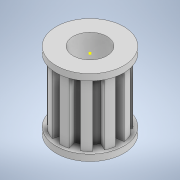
# Autodesk Inventor part: Pièce_moteur_courroie_test_1
Saved by Autodesk Inventor 2020.1 (Build 241239000, 239)
## iProperties
Created: 2019-07-26
Part Number: Pièce_moteur_courroie_test_1
Material: Générique
Document SubType Name: Modeling
Designer: marlo
Density: 1 g/cm^3
Appearance: Par défaut
Author: marlo
Autodesk Inventor part; units mm, degrees
ref_plane "YZ Plane" through (0, 0, 0) normal (1, 0, 0) x (0, 1, 0)
ref_plane "XZ Plane" through (0, 0, 0) normal (0, 1, 0) x (-1, 0, 0)
ref_plane "XY Plane" through (0, 0, 0) normal (0, 0, 1) x (1, 0, 0)
sketch "Esquisse2" plane through (0, 0, 0) normal (0, 1, 0) x (-1, 0, 0)
  circle A0 centre (0, 0) radius 7.2
  dimension "d0" = 14.4
  constraints: 1 centre point, 1 coincident
  measures "d0" diameter of A0
extrude "Extrusion1" add sketch "Esquisse2" along normal blind 15
sketch "Esquisse4" plane through (0, 15, 0) normal (0, 1, 0) x (1, 0, 0)
  circle A0 centre (0, 0) radius 7.2 projected
  circle A1 centre (0, 0) radius 7.2 projected
  arc A2 (-2, -6.9166) -> (0, -7.2) centre (0, 0) ccw
  arc A3 (-1.4444, -4.9954) -> (0, -5.2) centre (0, 0) ccw
  line L0 (-2, -6.9166) -> (-1.4444, -4.9954)
  line L1 (0, -7.2) -> (0, -5.2)
  line L2 (0, 0) -> (-4.1531, -9.129)
  arc A4 (-5.4277, -4.7308) -> (-3.9, -6.0523) centre (0, 0) ccw
  arc A5 (-3.92, -3.4167) -> (-2.8167, -4.3711) centre (0, 0) ccw
  line L3 (-3.9, -6.0523) -> (-2.8167, -4.3711)
  line L4 (-5.4277, -4.7308) -> (-3.92, -3.4167)
  line L5 (0, -6) -> (0, 5.5969) construction
  line L6 (0, 0) -> (-5.5895, -3.594)
  arc A6 (-6.5507, 2.988) -> (-7.1229, 1.0507) centre (0, 0) ccw
  arc A7 (-4.7311, 2.158) -> (-5.1443, 0.7589) centre (0, 0) ccw
  line L7 (-7.1229, 1.0507) -> (-5.1443, 0.7589)
  line L8 (-6.5507, 2.988) -> (-4.7311, 2.158)
  arc A8 (-7.125, -1.0366) -> (-6.5566, -2.975) centre (0, 0) ccw
  arc A9 (-5.1458, -0.7487) -> (-4.7353, -2.1486) centre (0, 0) ccw
  line L9 (-7.125, -1.0366) -> (-5.1458, -0.7487)
  line L10 (-6.5566, -2.975) -> (-4.7353, -2.1486)
  line L11 (-2, -6.9166) -> (-3.9, -6.0523) construction
  line L12 (-5.4277, -4.7308) -> (-6.5566, -2.975) construction
  line L13 (-2, -6.9166) -> (0, -7.2) construction
  line L14 (0, 0) -> (-5.7368, 3.7048)
  arc A10 (-3.888, 6.06) -> (-5.4183, 4.7415) centre (0, 0) ccw
  line L15 (-5.4183, 4.7415) -> (-3.9132, 3.4244)
  line L16 (-3.888, 6.06) -> (-2.808, 4.3767)
  arc A11 (-2.808, 4.3767) -> (-3.9132, 3.4244) centre (0, 0) ccw
  line L17 (-1.9863, 6.9206) -> (-1.4345, 4.9982)
  arc A12 (0.0143, 7.2) -> (-1.9863, 6.9206) centre (0, 0) ccw
  arc A13 (0.0103, 5.2) -> (-1.4345, 4.9982) centre (0, 0) ccw
  line L18 (0.0143, 7.2) -> (0.0103, 5.2)
  line L19 (-6.5507, 2.988) -> (-5.4183, 4.7415) construction
  line L20 (0, 0) -> (1.7786, 11.975)
  arc A14 (1.9726, -6.9245) -> (3.8184, -6.1041) centre (0, 0) ccw
  arc A15 (1.4246, -5.001) -> (2.7578, -4.4085) centre (0, 0) ccw
  line L21 (1.9726, -6.9245) -> (1.4246, -5.001)
  line L22 (3.8184, -6.1041) -> (2.7578, -4.4085)
  arc A16 (7.1208, -1.0648) -> (7.1364, 0.9551) centre (0, 0) ccw
  line L23 (7.1364, 0.9551) -> (5.154, 0.6898)
  line L24 (7.1208, -1.0648) -> (5.1428, -0.7691)
  arc A17 (5.1428, -0.7691) -> (5.154, 0.6898) centre (0, 0) ccw
  line L25 (6.5161, -3.0627) -> (4.7061, -2.212)
  arc A18 (5.4089, -4.7522) -> (6.5161, -3.0627) centre (0, 0) ccw
  arc A19 (3.9064, -3.4322) -> (4.7061, -2.212) centre (0, 0) ccw
  line L26 (5.4089, -4.7522) -> (3.9064, -3.4322)
  line L27 (3.8184, -6.1041) -> (5.4089, -4.7522) construction
  line L28 (2.079, 6.8933) -> (1.5015, 4.9785)
  arc A20 (2.8253, 4.3655) -> (1.5015, 4.9785) centre (0, 0) ccw
  line L29 (3.912, 6.0445) -> (2.8253, 4.3655)
  arc A21 (3.912, 6.0445) -> (2.079, 6.8933) centre (0, 0) ccw
  arc A22 (4.7396, 2.1392) -> (3.9588, 3.3716) centre (0, 0) ccw
  line L30 (5.4815, 4.6684) -> (3.9588, 3.3716)
  line L31 (6.5625, 2.962) -> (4.7396, 2.1392)
  arc A23 (6.5625, 2.962) -> (5.4815, 4.6684) centre (0, 0) ccw
  line L32 (7.1364, 0.9551) -> (6.5625, 2.962) construction
  line L33 (0.0143, 7.2) -> (2.079, 6.8933) construction
  point P0 (3.8184, -6.1041)
  point P1 (6.5161, -3.0627)
  point P2 (7.1208, -1.0648)
  point P3 (7.1364, 0.9551)
  point P4 (5.4815, 4.6684)
  point P5 (2.079, 6.8933)
  point P6 (-6.5507, 2.988)
  point P7 (-7.1229, 1.0507)
  point P8 (-6.5566, -2.975)
  point P9 (-2, -6.9166)
  point P10 (0, -7.2)
  point P11 (-5.4277, -4.7308)
  point P12 (-3.9, -6.0523)
  dimension "d13" = 2
  dimension "d14" = 2
  dimension "d16" = 1.9
  constraints: 68 end point, 46 point on circle, 40 symmetric about line, 22 centre point, 4 equal length, 2 point on line, 2 vertical, 1 coincident, 20 other
  measures "d13" radial gap between concentric circles of A0 A3
  measures "d14" horizontal distance of L0.start L1.start
  measures "d16" horizontal distance of L0.start L3.start
extrude "Extrusion2" cut sketch "Esquisse4" against normal through all contours A0 L24 A17 L23 | L31 A22 L30 A0 | A0 L26 A19 L25 | L29 A20 L28 A0 | A0 L21 A15 L22 | A0 L0 A3 L1 | L18 A13 L17 A0 | L16 A11 L15 A0 | A0 L4 A5 L3 | L8 A7 L7 A0 | A0 L9 A9 L10
sketch "Esquisse5" plane through (0, 15, 0) normal (0, 1, 0) x (1, 0, 0)
  point P0 (0, 0)
sketch "Esquisse6" plane through (0, 15, 0) normal (0, 1, 0) x (1, 0, 0)
  circle A0 centre (0, 0) radius 8
  dimension "d19" = 16
  constraints: 1 centre point, 1 coincident
  measures "d19" diameter of A0
extrude "Extrusion3" add sketch "Esquisse6" along normal blind 1.5
sketch "Esquisse7" plane through (0, 0, 0) normal (0, -1, 0) x (1, 0, 0)
  circle A0 centre (0, 0) radius 8
  constraints: 1 centre point, 1 coincident
extrude "Extrusion4" add sketch "Esquisse7" along normal blind 1.5
sketch "Esquisse8" plane through (0, 16.5, 0) normal (0, 1, 0) x (1, 0, 0)
  circle A0 centre (0, 0) radius 4
  dimension "d24" = 8
  constraints: 1 centre point, 1 coincident
  measures "d24" diameter of A0
extrude "Extrusion5" cut sketch "Esquisse8" against normal through all
